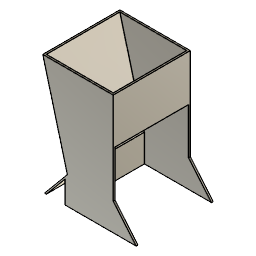
IMP Filter Funnel (Autodesk Fusion 360 design; units mm, degrees)
part number: 2026-02-27-22-43-34-164
Autodesk Fusion 360 part; units mm, degrees
note: some values were not read from the file. Set by a fixed rule: which sketch regions a step uses.
sketch "Sketch1" plane through (0, 0, 0) normal (0, 1, 0) x (1, 0, 0)
  line L0 (0, 0) -> (0, -60)
  line L1 (0, 0) -> (100, 0) construction
  line L2 (100, 0) -> (100, -60) construction
  line L3 (100, -60) -> (0, -60) construction
  line L4 (0, -60) -> (0, 0) construction
  line L5 (100, -60) -> (100, -260)
  line L6 (0, -60) -> (207.1474, -60) construction
  line L7 (0, -60) -> (0, -260) construction
  line L8 (0, -260) -> (-150, -260) construction
  line L9 (0, -60) -> (-53.5898, -260)
  line L10 (0, -60) -> (207.0552, -60) construction
  line L11 (100, -260) -> (-53.5898, -260)
  line L12 (0, 0) -> (100, 0)
  line L13 (100, 0) -> (150, 0)
  line L14 (150, 0) -> (100, -60)
  line L15 (0, 0) -> (-50, 0) construction
  line L16 (-50, 0) -> (-50, -60) construction
  line L17 (-50, -60) -> (0, -60) construction
  line L18 (0, -60) -> (0, 0) construction
  line L19 (-50, -60) -> (0, 0) construction
  line L20 (-50, 0) -> (0, -60) construction
  line L21 (-50, 0) -> (-50, 20) construction
  line L22 (-50, 0) -> (-50, 5) construction
  line L23 (0, -60) -> (0, -55) construction
  line L24 (0, -60) -> (0, -55)
  line L25 (-50, 0) -> (-50, 5)
  line L26 (-50, 0) -> (0, -60)
  line L27 (-50, 5) -> (0, -55) construction
  line L28 (-50, 0) -> (-45.8333, 0)
  line L29 (-45.8333, 0) -> (0, -55)
  line L30 (0, 0) -> (-5, 0) construction
  line L31 (-5, 0) -> (-5, -49)
  line L32 (-5, 0) -> (0, 0)
  dimension "d2" = 60
  dimension "d3" = 200
  dimension "d17" = 105
  dimension "d26" = 50
  dimension "d27" = 60
  dimension "d28" = 5
  dimension "d29" = 90
  constraint coincident L0.start L1.start
  constraint horizontal L1
  constraint vertical L2
  constraint horizontal L3
  constraint vertical L4
  constraint perpendicular L3 L5
  constraint horizontal L6
  constraint perpendicular L6 L7
  constraint perpendicular L7 L8
  constraint horizontal L10
  constraint coincident L8 L9.end
  constraint perpendicular L7 L11
  constraint perpendicular L2 L13
  constraint horizontal L15
  constraint vertical L16
  constraint horizontal L17
  constraint vertical L18
  constraint perpendicular L15 L21
  constraint perpendicular L15 L22
  constraint coincident L18 L23.end
  constraint perpendicular L6 L23
  constraint parallel L26 L27
  constraint coincident L15 L28.end
  constraint coincident L27 L28.end
  constraint coincident L15 L30.end
  constraint coincident L27 L31.end
  measures "d2" distance of L0.start L0.end
  measures "d3" distance of L2.end L5.end
  measures "d17" angle of L9 L10
  measures "d26" distance of L0.start L15.end
  measures "d27" distance of L0.start L0.end
  measures "d28" distance of L15.end L22.end
  measures "d29" angle of L30 L31
extrude "Extrude1" add sketch "Sketch1" along normal blind 4 contours L0 L5 L9 L11 L12 L13 L14 L24 makes body 1
sketch "Sketch2" plane through (0, 0, 0) normal (0, 0, 1) x (1, 0, 0)
  line L0 (0, 0) -> (0, -80) construction
  line L1 (0, 0) -> (0, 80) construction
  dimension "d7" = 80
  dimension "d8" = 80
  constraint coincident L0.start L1.start
  constraint vertical L0
  constraint parallel L0 L1
  measures "d7" distance of L0.start L0.end
  measures "d8" distance of L0.start L1.end
move_body "Move1" bodies 1 to x (1, 0, 0) y (0, 1, 0) z (0, 0, 1) at (0, 80, 0)
pattern_linear "R-Pattern1" count 2 spacing 164 along (0, -1, 0) of bodies 1 makes body 2
sketch "Sketch3" plane through (0, -84, 0) normal (0, -1, 0) x (1, 0, 0)
  line L0 (0, 60) -> (0, 0)
  line L1 (100, 60) -> (100, 260)
  line L2 (0, 0) -> (4, 0)
  line L3 (4, 0) -> (4, 60)
  line L4 (4, 60) -> (0, 60)
  line L5 (0, 60) -> (0, 0)
  line L6 (100, 260) -> (-53.5898, 260)
  line L7 (-53.5898, 260) -> (0, 60)
  line L8 (0, 0) -> (150, 0)
  line L9 (150, 0) -> (100, 60)
  dimension "d13" = 4
  dimension "d14" = 60
  constraint horizontal L2
  constraint vertical L3
  constraint horizontal L4
  constraint vertical L5
  constraint coincident L0.end L2.start
  measures "d13" distance of L0.end L2.end
  measures "d14" distance of L0.end L0.start
extrude "Extrude2" add sketch "Sketch3" against normal blind 168 contours L0 L2 L3 L4 L5 L8 bodies 1 2
sketch "Sketch4" plane through (0, -84, 0) normal (0, -1, 0) x (1, 0, 0)
  line L0 (0, 0) -> (150, 0)
  line L1 (100, 60) -> (100, 260)
  line L2 (100, 260) -> (-53.5898, 260)
  line L3 (-53.5898, 260) -> (0, 60)
  line L4 (0, 60) -> (0, 0)
  line L5 (0, 60) -> (0, 260) construction
  line L6 (-53.5898, 260) -> (0, 260) construction
  line L7 (-53.5898, 260) -> (-49.5898, 260) construction
  line L8 (0, 60) -> (100, 60) construction
  line L9 (0, 60) -> (4, 60) construction
  line L10 (-49.5898, 260) -> (4, 60)
  line L11 (4, 60) -> (0, 60)
  line L12 (150, 0) -> (100, 60)
  dimension "d18" = 4
  dimension "d19" = 4
  constraint coincident L3.end L4.start
  constraint coincident L2 L5.end
  constraint perpendicular L2 L5
  constraint coincident L2.end L3.start
  constraint parallel L6 L7
  constraint coincident L1.start L8.end
  constraint perpendicular L5 L9
  measures "d18" distance of L2.end L7.end
  measures "d19" distance of L3.end L9.end
extrude "Extrude3" add sketch "Sketch4" against normal blind 168 contours L2 L3 L10 L11 bodies 1
sketch "Sketch5" plane through (0, -84, 0) normal (0, -1, 0) x (1, 0, 0)
  line L0 (100, 260) -> (-53.5898, 260)
  line L1 (-53.5898, 260) -> (0, 60)
  line L2 (0, 60) -> (0, 0)
  line L3 (0, 0) -> (150, 0)
  line L4 (100, 60) -> (100, 260)
  line L5 (100, 260) -> (96, 260)
  line L6 (96, 260) -> (96, 160)
  line L7 (96, 160) -> (100, 160)
  line L8 (100, 160) -> (100, 260)
  line L9 (150, 0) -> (100, 60)
  dimension "d22" = 4
  dimension "d23" = 100
  constraint horizontal L5
  constraint vertical L6
  constraint horizontal L7
  constraint vertical L8
  constraint coincident L0.start L4.end
  measures "d22" distance of L0.start L5.end
  measures "d23" distance of L0.start L7.end
extrude "Extrude4" add sketch "Sketch5" against normal blind 168 contours L0 L4 L5 L6 L7 L8 bodies 1
extrude "Extrude5" add sketch "Sketch1" along normal mid plane 168 contours L0 L29 L31 L32 | L0 L24 L26 L28 L29 bodies 1
